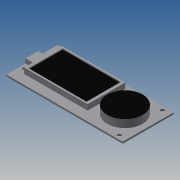
# Autodesk Inventor part: miniviki
Saved by Autodesk Inventor 2013 (Build 170138000, 138)
## iProperties
Created: 2017-04-06
Part Number: miniviki
Material: Generic
Document SubType Name: Modeling
Designer: employee
Density: 1 g/cm^3
Author: employee
Autodesk Inventor part; units mm, degrees
ref_plane "YZ Plane" through (0, 0, 0) normal (1, 0, 0) x (0, 1, 0)
ref_plane "XZ Plane" through (0, 0, 0) normal (0, 1, 0) x (-1, 0, 0)
ref_plane "XY Plane" through (0, 0, 0) normal (0, 0, 1) x (1, 0, 0)
sketch "Sketch1" plane through (0, 0, 0) normal (0, 0, 1) x (1, 0, 0)
  line L0 (-52.6, 23) -> (52.6, 23)
  line L1 (52.6, 23) -> (52.6, -23)
  line L2 (52.6, -23) -> (-52.6, -23)
  line L3 (-52.6, -23) -> (-52.6, 23)
  point P0 (0, 0)
  point P1 (-52.6, 0)
  point P2 (0, 23)
  dimension "d0" = 105.2
  dimension "d2" = 46
  constraints: 8 end point, 2 midpoint, 2 parallel, 1 horizontal, 1 horizontal alignment, 1 perpendicular, 1 vertical alignment
  measures "d0" distance of L1.end L2.end
  measures "d2" distance of L2.end L0.start
extrude "Extrusion1" add sketch "Sketch1" along normal blind 1.6
sketch "Sketch2" plane through (0, 0, 1.6) normal (0, 0, 1) x (1, 0, 0)
  line L0 (-52.6, -23) -> (52.6, -23) projected
  line L1 (52.6, -23) -> (52.6, 23) projected
  line L2 (-45.1, 19.5) -> (12.4, 19.5)
  line L3 (12.4, 19.5) -> (12.4, -14.5)
  line L4 (12.4, -14.5) -> (-45.1, -14.5)
  line L5 (-45.1, -14.5) -> (-45.1, 19.5)
  circle A0 centre (31.6, 0) radius 16
  line L6 (31.6, 0) -> (31.6, -16)
  line L7 (31.6, 0) -> (31.6, 16)
  line L8 (52.6, 23) -> (-52.6, 23) projected
  line L9 (-52.6, 23) -> (-52.6, -23) projected
  point P0 (0, 0)
  dimension "d5" = 57.5
  dimension "d7" = 34
  dimension "d8" = 32
  dimension "d9" = 21
  dimension "d10" = 23
  dimension "d13" = 3.5
  dimension "d14" = 7.5
  constraints: 12 end point, 3 parallel, 2 point on circle, 1 centre point, 1 collinear, 1 horizontal, 1 perpendicular
  measures "d5" distance of L2.start L2.end
  measures "d7" distance of L4.end L2.start
  measures "d8" diameter of A0
  measures "d9" distance from line of L1 L6.start
  measures "d10" distance from line of L6.start L0
  measures "d13" distance between parallel lines of L8 L2
  measures "d14" distance between parallel lines of L5 L9
extrude "Extrusion2" add sketch "Sketch2" along normal blind 7 contours L2 L3 L4 L5 | A0 L6 L7 | L7 L6 A0
sketch "Sketch3" plane through (0, 0, 8.6) normal (0, 0, 1) x (1, 0, 0)
  line L0 (12.4, 19.5) -> (-45.1, 19.5) projected
  line L1 (-45.1, 19.5) -> (-45.1, -14.5) projected
  line L2 (-45.1, -14.5) -> (12.4, -14.5) projected
  line L3 (12.4, -14.5) -> (12.4, 19.5) projected
  point P0 (0, 0)
extrude "Extrusion3" cut sketch "Sketch3" against normal blind 2
sketch "Sketch4" plane through (0, 0, 6.6) normal (0, 0, 1) x (1, 0, 0)
  line L0 (-45.1, 19.5) -> (12.4, 19.5) projected
  line L1 (-45.1, -14.5) -> (-45.1, 19.5) projected
  line L2 (-42.5865, 18.0138) -> (9.8865, 18.0138)
  line L3 (9.8865, 18.0138) -> (9.8865, -13.0138)
  line L4 (9.8865, -13.0138) -> (-42.5865, -13.0138)
  line L5 (-42.5865, -13.0138) -> (-42.5865, 18.0138)
  line L6 (-45.1, -14.5) -> (-42.5865, -13.0138) construction
  point P0 (0, 0)
  point P1 (-45.1, 2.5)
  point P2 (-42.5865, 2.5)
  point P3 (-16.35, 18.0138)
  point P4 (-16.35, 19.5)
  dimension "d21" = 60.96
  constraints: 10 end point, 4 midpoint, 2 parallel, 1 horizontal, 1 horizontal alignment, 1 perpendicular, 1 point on line, 1 vertical alignment
  measures "d21" distance of L2.end L4.end
extrude "Extrusion4" cut sketch "Sketch4" against normal blind 1
sketch "Sketch5" plane through (0, 0, 1.6) normal (0, 0, 1) x (1, 0, 0)
  line L0 (-52.6, 23) -> (-52.6, -23) projected
  line L1 (-52.6, -5.75) -> (-45.1, -5.75)
  line L2 (-45.1, -5.75) -> (-45.1, 5.75)
  line L3 (-45.1, 5.75) -> (-52.6, 5.75)
  line L4 (-52.6, 5.75) -> (-52.6, -5.75)
  line L5 (-45.1, -14.5) -> (-45.1, 19.5) projected
  point P0 (0, 0)
  point P1 (-45.1, 0)
  point P2 (-52.6, 0)
  dimension "d24" = 11.5
  constraints: 8 end point, 3 midpoint, 2 parallel, 2 point on line, 1 horizontal, 1 perpendicular
  measures "d24" distance between parallel lines of L3 L1
extrude "Extrusion5" add sketch "Sketch5" along normal blind 4
sketch "Sketch6" plane through (-52.6, -23, 0) normal (-1, 0, 0) x (0, 0, 1)
  line L0 (1.6, 17.25) -> (5.6, 17.25) projected
  line L1 (5.6, 28.75) -> (5.6, 17.25) projected
  line L2 (1.6, 28.75) -> (5.6, 28.75) projected
  line L3 (1.6, 46) -> (1.6, 28.75) projected
  line L4 (4.1, 28.55) -> (5.4, 28.55)
  line L5 (5.4, 28.55) -> (5.4, 17.45)
  line L6 (5.4, 17.45) -> (4.1, 17.45)
  line L7 (4.1, 17.45) -> (4.1, 28.55)
  point P0 (0, 23)
  dimension "d28" = 2.5
  dimension "d29" = 0.2
  dimension "d30" = 0.2
  dimension "d31" = 0.2
  constraints: 8 end point, 2 parallel, 1 horizontal, 1 perpendicular
  measures "d28" distance between parallel lines of L3 L7
  measures "d29" distance between parallel lines of L2 L4
  measures "d30" distance between parallel lines of L5 L1
  measures "d31" distance between parallel lines of L0 L6
extrude "Extrusion6" cut sketch "Sketch6" against normal up to surface (7.5 mm away)
sketch "Sketch7" plane through (0, 0, 1.6) normal (0, 0, 1) x (1, 0, 0)
  line L0 (52.6, -23) -> (52.6, 23) projected
  line L1 (-52.6, 23) -> (-52.6, 5.75) projected
  line L2 (-45.1, -14.5) -> (-45.1, -5.75) projected
  circle A0 centre (-48.85, -10.125) radius 1.75
  circle A1 centre (-48.85, 10.125) radius 1.75
  circle A2 centre (46.1, 19.5) radius 1.75
  circle A3 centre (46.1, -19.5) radius 1.75
  line L3 (-48.85, 10.125) -> (-48.85, -10.125) construction
  line L4 (46.1, 19.5) -> (46.1, -19.5) construction
  point P0 (0, 0)
  point P1 (52.6, 0)
  point P2 (-48.85, 0)
  point P3 (46.1, 0)
  point P4 (52.6, 0)
  point P5 (52.6, 0)
  dimension "d34" = 20.25
  dimension "d36" = 3.75
  dimension "d37" = 39
  dimension "d39" = 6.5
  dimension "d40" = 3.5
  constraints: 5 midpoint, 4 centre point, 4 end point, 3 equal radius, 2 horizontal alignment, 1 parallel, 1 vertical
  measures "d34" distance of L3.start L3.end
  measures "d36" distance between parallel lines of L3 L1
  measures "d37" distance of L4.start L4.end
  measures "d39" distance between parallel lines of L4 L0
  measures "d40" diameter of A1
extrude "Extrusion7" cut sketch "Sketch7" against normal through all
body "Solid1"
